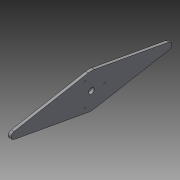
# Autodesk Inventor part: RibSimple
Saved by Autodesk Inventor 2014 SP1 (Build 180222100, 222)
## iProperties
Created: 2014-11-10
Part Number: RibSimple
Material: Generic
Document SubType Name: Modeling
Designer: rawrdong
Density: 1 g/cm^3
Appearance: Default
Author: rawrdong
Autodesk Inventor part; units mm, degrees
ref_plane "YZ Plane" through (0, 0, 0) normal (1, 0, 0) x (0, 1, 0)
ref_plane "XZ Plane" through (0, 0, 0) normal (0, 1, 0) x (-1, 0, 0)
ref_plane "XY Plane" through (0, 0, 0) normal (0, 0, 1) x (1, 0, 0)
sketch "Sketch1" plane through (0, 0, 0) normal (1, 0, 0) x (0, 1, 0)
  line L0 (-128.1, 0) -> (128.1, 0) projected
  line L1 (0, -28) -> (0, 28) construction
  arc A0 (88.2166, -3.9353) -> (88.2166, 3.9353) centre (87.5, 0) ccw
  arc A1 (-88.2166, 3.9353) -> (-88.2166, -3.9353) centre (-87.5, 0) ccw
  line L2 (-88.2166, 3.9353) -> (0, 20)
  line L3 (0, 20) -> (88.2166, 3.9353)
  line L4 (88.2166, -3.9353) -> (0, -20)
  line L5 (-88.2166, -3.9353) -> (0, -20)
  circle A2 centre (0, 0) radius 3.175
  circle A3 centre (15, 0) radius 0.75
  line L6 (15, 0) -> (-7.5, -12.9904) construction
  line L7 (-7.5, -12.9904) -> (-7.5, 12.9904) construction
  line L8 (-7.5, 12.9904) -> (15, 0) construction
  circle A4 centre (-7.5, 12.9904) radius 0.75
  circle A5 centre (-7.5, -12.9904) radius 0.75
  circle A6 centre (0, 0) radius 15 construction
  dimension "d7" = 30
  dimension "d0" = 8
  dimension "d1" = 175
  dimension "d3" = 6.35
  dimension "d4" = 1.5
  dimension "d11" = 40
  constraints: 14 end point, 6 centre point, 5 coincident, 5 point on line, 4 point on circle, 4 tangent, 3 equal radius, 1 parallel, 1 symmetric about line, 10 other
  measures "d0" diameter of A1
  measures "d1" distance of A0.centre A1.centre
  measures "d3" diameter of A2
  measures "d4" diameter of A3
  measures "d11" distance of L2.end L4.end
extrude "Extrusion1" add sketch "Sketch1" along normal blind 3.2 contours A1 L2 L3 A0 L0 A3 A2 | L0 A2 A3 A0 L4 L5 A1
fillet "Fillet1" radius 20 2 edges at (1.6, 0, 20) (1.6, 0, -20)
sketch "Sketch3" plane through (3.2, 0, 0) normal (1, 0, 0) x (0, 0, -1)
  line L0 (-7.7286, 24.361) -> (0, 66.8014)
  line L1 (0, 66.8014) -> (7.7286, 24.361)
  line L2 (8.0286, -24.361) -> (0, -68.4486)
  line L3 (0, -68.4486) -> (-8.0286, -24.361)
  line L4 (-7.7286, 24.361) -> (7.7286, 24.361)
  line L5 (-8.0286, -24.361) -> (8.0286, -24.361)
  line L6 (27.5395, 0) -> (-27.5395, 0) projected
  constraints: 12 end point, 1 horizontal, 1 parallel, 1 other
sketch "Sketch2" plane through (3.2, 0, 0) normal (1, 0, 0) x (0, 0, -1)
  circle A0 centre (0, 0) radius 3.175 projected
  circle A1 centre (0, 0) radius 3.048
  dimension "d13" = 6.096
  constraints: 1 centre point, 1 coincident
  measures "d13" diameter of A1
body "Solid1"
